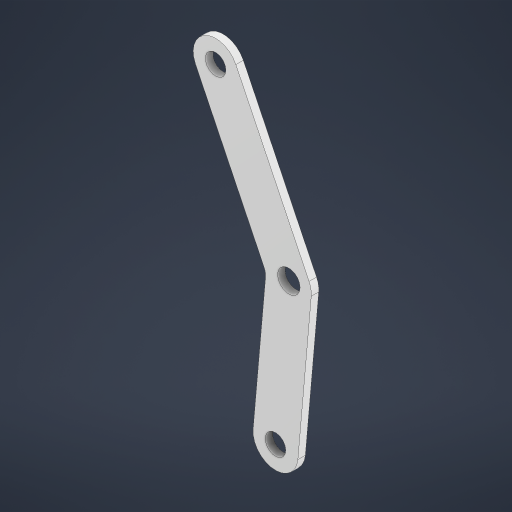
# Autodesk Inventor part: pneumaticintake
Saved by Autodesk Inventor 2023 (Build 270158000, 158)
## iProperties
Created: 2023-08-12
Part Number: pneumaticintake
Material: Generic
Document SubType Name: Modeling
Designer: srbel
Density: 1 g/cm^3
Appearance: Smooth - White
Author: srbel
Autodesk Inventor part; units mm, degrees
ref_plane "YZ Plane" through (0, 0, 0) normal (1, 0, 0) x (0, 1, 0)
ref_plane "XZ Plane" through (0, 0, 0) normal (0, 1, 0) x (-1, 0, 0)
ref_plane "XY Plane" through (0, 0, 0) normal (0, 0, 1) x (1, 0, 0)
sketch "Sketch1" plane through (0, 0, 0) normal (0, 0, 1) x (1, 0, 0)
  circle A0 centre (57.15, 5.5563) radius 2.1844
  circle A1 centre (72.6846, -26.511) radius 2.39
  circle A2 centre (69.85, -57.9437) radius 2.1844
  circle A3 centre (69.85, -57.9437) radius 2.1844
  arc A4 (65.1067, -57.5159) -> (74.5933, -58.3714) centre (69.85, -57.9437) ccw
  arc A5 (77.4279, -26.9388) -> (76.9707, -24.4347) centre (72.6846, -26.511) ccw
  circle A6 centre (57.15, 5.5563) radius 2.1844
  arc A7 (61.4361, 7.6326) -> (52.8639, 3.4799) centre (57.15, 5.5563) ccw
  circle A8 centre (72.6846, -26.511) radius 2.39
  line L0 (52.8639, 3.4799) -> (67.4389, -26.6063)
  line L1 (67.7437, -28.2757) -> (65.1067, -57.5159)
  line L2 (77.4279, -26.9388) -> (74.5933, -58.3714)
  line L3 (61.4361, 7.6326) -> (76.9707, -24.4347)
  arc A9 (67.7437, -28.2757) -> (67.4389, -26.6063) centre (64.5815, -27.9905) ccw
  point P0 (0, 0)
  dimension "d0" = 9.525
  dimension "d1" = 9.525
  dimension "d2" = 9.525
  dimension "d3" = 3.175
  constraints: 10 centre point, 10 tangent, 8 end point, 8 point on circle, 5 coincident, 3 concentric, 5 other
  measures "d0" diameter of A4
  measures "d1" diameter of A5
  measures "d2" diameter of A7
  measures "d3" radius of A9
extrude "Extrusion1" add sketch "Sketch1" along normal blind 1.5875
body "Solid1"
